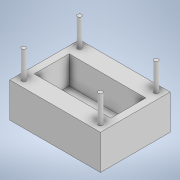
# Autodesk Inventor part: bottom
Saved by Autodesk Inventor 2022 (Build 260153000, 153)
## iProperties
Created: 2024-03-25
Part Number: bottom
Material: Generic
Document SubType Name: Modeling
Designer: subin
Density: 1 g/cm^3
Appearance: Default
Author: subin
Autodesk Inventor part; units mm, degrees
ref_plane "YZ Plane" through (0, 0, 0) normal (1, 0, 0) x (0, 1, 0)
ref_plane "XZ Plane" through (0, 0, 0) normal (0, 1, 0) x (-1, 0, 0)
ref_plane "XY Plane" through (0, 0, 0) normal (0, 0, 1) x (1, 0, 0)
sketch "Sketch1" plane through (0, 0, 0) normal (0, 1, 0) x (-1, 0, 0)
  line L0 (0, 0) -> (-130, 0)
  line L1 (-130, 0) -> (-130, -100)
  line L2 (-130, -100) -> (0, -100)
  line L3 (0, -100) -> (0, 0)
  dimension "d0" = 130
  dimension "d1" = 100
  constraints: 8 end point, 2 parallel, 1 horizontal, 1 perpendicular
  measures "d0" distance of L2.end L1.end
  measures "d1" distance between parallel lines of L2 L0
extrude "Extrusion1" add sketch "Sketch1" along normal blind 10
sketch "Sketch2" plane through (0, 10, 0) normal (0, 1, 0) x (1, 0, 0)
  line L0 (10, 25) -> (120, 25)
  line L1 (120, 25) -> (120, 75)
  line L2 (120, 75) -> (10, 75)
  line L3 (10, 75) -> (10, 25)
  line L4 (130, 100) -> (0, 100) projected
  line L5 (130, 0) -> (130, 100) projected
  line L6 (0, 100) -> (0, 0) projected
  line L7 (0, 0) -> (130, 0) projected
  dimension "d4" = 25
  dimension "d5" = 10
  dimension "d6" = 10
  dimension "d7" = 25
  constraints: 8 end point, 2 parallel, 1 horizontal, 1 perpendicular
  measures "d4" distance between parallel lines of L4 L2
  measures "d5" distance between parallel lines of L5 L1
  measures "d6" distance between parallel lines of L6 L3
  measures "d7" distance between parallel lines of L7 L0
extrude "Extrusion2" add sketch "Sketch2" along normal blind 40
sketch "Sketch3" plane through (0, 50, 0) normal (0, 1, 0) x (1, 0, 0)
  circle A0 centre (10, 90) radius 3
  line L0 (130, 100) -> (0, 100) projected
  line L1 (0, 100) -> (0, 0) projected
  line L2 (130, 0) -> (130, 100) projected
  line L3 (130, 100) -> (0, 100) projected
  line L4 (65, 100) -> (65, 0)
  line L5 (0, 0) -> (130, 0) projected
  line L6 (0, 100) -> (0, 0) projected
  line L7 (0, 50) -> (130, 50)
  circle A1 centre (120, 90) radius 3
  circle A2 centre (10, 10) radius 3
  line L8 (130, 0) -> (0, 0)
  line L9 (130, 0) -> (0, 0)
  circle A3 centre (120, 10) radius 3
  dimension "d10" = 6
  dimension "d11" = 10
  dimension "d12" = 10
  constraints: 8 end point, 4 centre point, 4 midpoint, 3 symmetric about line, 3 other
  measures "d10" diameter of A0
  measures "d11" distance from line of L0 A0.centre
  measures "d12" distance from line of L1 A0.centre
extrude "Extrusion3" add sketch "Sketch3" along normal blind 40 contours A0 | A1 | A2 | A3
body "Solid1"
